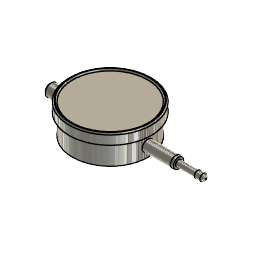
HALS-Total (Autodesk Fusion 360 archive; units mm, degrees)
design "DIAL-INDICATOR"
Autodesk Fusion 360 part; units mm, degrees
cylinder "CylinderPrimitive1" add diameter 55.25 height 15 placed x (1, 0, 0) y (0, 1, 0) z (0, 0, 1) at (0, 0, 0) makes body 1
cylinder "CylinderPrimitive2" add diameter 60 height 7.5 placed x (1, 0, 0) y (0, 1, 0) z (0, 0, 1) at (0, 0, 15) bodies 1
cylinder "CylinderPrimitive3" add diameter 8 height 85 placed x (0, 0, -1) y (0, 1, 0) z (1, 0, 0) at (0, 0, 0) separate body makes body 2
move_body "Move1" bodies 2 to x (1, 0, 0) y (0, 1, 0) z (0, 0, 1) at (-35, 0, 7.5)
cylinder "CylinderPrimitive4" add diameter 4.5 height 14 placed x (0, 0, -1) y (0, 1, 0) z (1, 0, 0) at (50, 0, 7.5) bodies 2
cylinder "CylinderPrimitive5" add diameter 5 height 6 placed x (0, 0, -1) y (0, 1, 0) z (1, 0, 0) at (64, 0, 7.5) bodies 2
chamfer "Chamfer1" distance 0.25 distance2 2 1 edges at (50, -1.4465, 11.2293) measured on face at (50, -0.1987, 4.0982) on bodies 2
fillet "Fillet1" radius 2 1 edges at (70, -0.904, 9.8308) on bodies 2
cylinder "CylinderPrimitive6" add diameter 9 height 9 placed x (0, 0, 1) y (0, 1, 0) z (-1, 0, 0) at (-35, 0, 7.5) bodies 2
fillet "Fillet2" radius 1 1 edges at (-44, -1.6273, 3.3045) on bodies 2
combine "Combine1" operation add target body 1 tool bodies 2
chamfer "Chamfer2" distance 1 distance2 1 1 edges at (-27.9698, -10.8485, 22.5) measured on face at (7.6631, 11.2397, 22.5) on bodies 1
cylinder "CylinderPrimitive7" cut diameter 54.918 height -1 placed x (1, 0, 0) y (0, 1, 0) z (0, 0, 1) at (0, 0, 22.5) bodies 1
chamfer "Chamfer3" distance 1 distance2 1 1 edges at (-9.9296, -25.6008, 22.5) measured on face at (28.3784, -1.4407, 22.5) on bodies 1
cylinder "CylinderPrimitive8" add diameter 9.5 height -34 placed x (0, 0, -1) y (0, 1, 0) z (1, 0, 0) at (0, 0, 0) separate body makes body 3
move_body "Move2" bodies 3 to x (0.707107, -0.707107, 0) y (0.707107, 0.707107, 0) z (0, 0, 1) at (0, 0, 0)
fillet "Fillet3" offset 2 second offset 1 tangency weight 0.5 1 edges at (-27.1731, 20.9102, 1.7177) measured on face at (-24.6363, 23.447, -0.2997) on bodies 3
move_body "Move3" bodies 3 to x (1, 0, 0) y (0, 1, 0) z (0, 0, 1) at (0, 0, 7.5)
combine "Combine2" operation add target body 1 tool bodies 3
named bodies: "DIAL-INDICATOR"

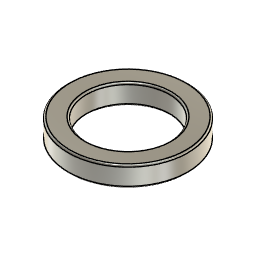
design "Kogellager 72x50x12 6910-2RS"
Autodesk Fusion 360 part; units mm, degrees
cylinder "CylinderPrimitive1" add diameter 72 height 12 placed x (1, 0, 0) y (0, 1, 0) z (0, 0, 1) at (0, 0, 0)
hole "Hole1" at (0, 0, 12) direction (0, 0, -1) diameter 50 depth 12 tip angle 180
fillet "Fillet1" radius 1 4 edges at (-33.5638, -13.0182, 12) (-23.3082, 9.0404, 12) (-33.5638, 13.0182, 0) (-23.3082, -9.0404, 0)
